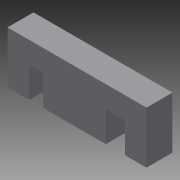
# Autodesk Inventor part: damping_blocker
Saved by Autodesk Inventor 2015 SP1 (Build 190203100, 203)
## iProperties
Created: 2015-08-28
Part Number: damping_blocker
Material: Generic
Document SubType Name: Modeling
Designer: Alexandre Cherpillod
Density: 1 g/cm^3
Appearance: Default
Author: Alexandre Cherpillod
Autodesk Inventor part; units mm, degrees
ref_plane "YZ Plane" through (0, 0, 0) normal (1, 0, 0) x (0, 1, 0)
ref_plane "XZ Plane" through (0, 0, 0) normal (0, 1, 0) x (-1, 0, 0)
ref_plane "XY Plane" through (0, 0, 0) normal (0, 0, 1) x (1, 0, 0)
sketch "Sketch1" plane through (0, 0, 0) normal (0, 1, 0) x (-1, 0, 0)
  line L0 (0, 0) -> (16.05, 0)
  line L1 (16.05, 0) -> (16.05, -6)
  line L2 (16.05, -6) -> (13.55, -6)
  line L3 (13.55, -6) -> (13.55, -2.5)
  line L4 (13.55, -2.5) -> (11.9, -2.5)
  line L5 (11.9, -2.5) -> (11.9, -6)
  line L6 (11.9, -6) -> (4.7, -6)
  line L7 (4.7, -6) -> (4.7, -2.5)
  line L8 (4.7, -2.5) -> (2.5, -2.5)
  line L9 (2.5, -2.5) -> (2.5, -6)
  line L10 (2.5, -6) -> (0, -6)
  line L11 (0, -6) -> (0, 0)
  dimension "d1" = 7.2
  dimension "d2" = 1.65
  dimension "d3" = 2.2
  dimension "d4" = 2.5
  dimension "d5" = 2.5
  dimension "d7" = 3.5
  dimension "d8" = 2.5
  constraints: 24 end point, 8 perpendicular, 6 point on line, 1 horizontal
  measures "d1" distance of L5.end L6.end
  measures "d2" distance of L3.end L4.end
  measures "d3" distance of L7.end L8.end
  measures "d4" distance of L1.end L2.end
  measures "d5" distance of L9.end L10.end
  measures "d7" distance of L8.end L9.end
  measures "d8" distance between parallel lines of L0 L4
extrude "Extrusion1" add sketch "Sketch1" along normal blind 3
body "Solid1"
